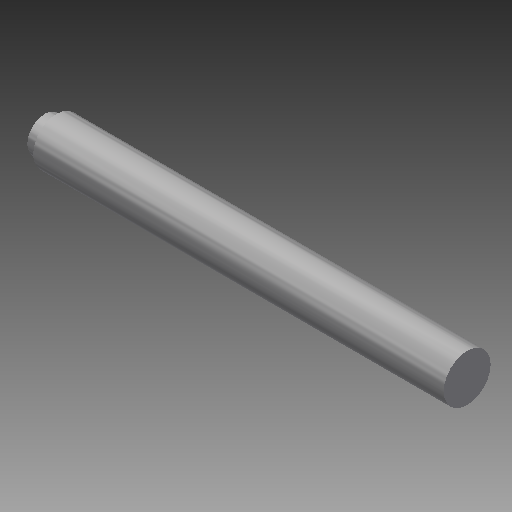
# Autodesk Inventor part: Shaft
Saved by Autodesk Inventor 2019 (Build 230136000, 136)
## iProperties
Created: 2019-10-31
Part Number: Shaft
Material: Steel
Document SubType Name: Modeling
Designer: Mark
Density: 1 g/cm^3
Appearance: Steel
CustomPartVersion: 1
Author: Mark
Autodesk Inventor part; units mm, degrees
ref_plane "Start Plane" through (0, 0, 0) normal (1, 0, 0) x (0, 1, 0)
ref_plane "XZ Plane" through (0, 0, 0) normal (0, 1, 0) x (-1, 0, 0)
ref_plane "XY Plane" through (0, 0, 0) normal (0, 0, 1) x (1, 0, 0)
sketch "Main Sketch" plane through (0, 0, 0) normal (0, 0, 1) x (1, 0, 0)
  line L0 (0, 0) -> (180, 0)
  line L1 (0, 0) -> (0, 7.5)
  line L2 (0, 7.5) -> (5, 7.5)
  line L3 (5, 7.5) -> (5, 10)
  line L4 (180, 10) -> (180, 0)
  line L5 (5, 10) -> (180, 10)
  dimension "d3" = 15
  dimension "d4" = 20
  constraints: 12 end point, 3 vertical, 1 horizontal
  measures "d3" diameter of L2 L0
  measures "d4" diameter of L5 L0
revolve "Revolution1" add sketch "Main Sketch" angle 360 about axis through (0, 0, 0) along (1, 0, 0)
body "Solid1"
